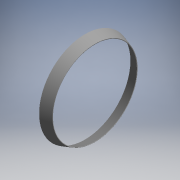
# Autodesk Inventor part: T4DB 170_cage
Saved by Autodesk Inventor 2017.3 (Build 213256000, 256)
## iProperties
Part Number: T4DB 170_cage
Material: Generic
Catalog Web Link: www.cadenas.de
Description: BT1_001_101_cage-Tapered roller bearings, single row
Vendor: SKF
Document SubType Name: Modeling
Designer: partserver
Manufacturer: SKF
Mass: 17.2348 g
Surface Area: 356.766 cm^2
Volume: 17.2348 cm^3
Density: 1 g/cm^3
Appearance: PSOLRGB-175-175-175
Category: PARTsolutions
Company: SKF
Title: T4DB 170_cage
Author: Cadenas PARTsolutions
Comments: Tapered roller bearings, single row
PSOL_IDENT_0: {$CADENAS_DATA\23d-libs\skf\bearings_units_and_housings\roller_bearings\tapered_roller_bearings\tape
PSOL_IDENT_1: red_roller_bearings_single_row\parts\bt1_001_101_cage.prj},178 {VTYP=3D},{NB=T4DB 170_cage},{LINA=T4
PSOL_IDENT_2: DB 170_cage},{NN=BT1_001_101_cage},{DATE=23.12.2020 07:01:43},{GEOMDATE=22.10.2020 06:54:36},{VERSIO
PSOL_IDENT_3: N=},{LINEID=4320},{WBVAR=},{WBNUMERIC=}  {NB=T4DB 170_cage},{LINA=T4DB 170_cage},{KT=DUMMY},{DESIGNA
PSOL_IDENT_4: TION=T4DB 170},{DD=170.000},{D=230.000},{T=32.000},{DD1=197.5000},{D1=MIN},{ALPHA=17.100},{RANGLE=2.
PSOL_IDENT_5: 500},{IRA=14.600},{B=30.000},{C=23.000},{C1=MIN},{R12=3.0},{R34=3.0},{AA=44.29541},{PITCH=200.033},{
PSOL_IDENT_6: DW=16.450},{LW=21.500},{DDAMAX=182},{DDAMIN=184.5},{DAMIN=215},{DAMAX=216.0},{DBMIN=223},{CA=6},{CB=
PSOL_IDENT_7: 9.0},{RA=3.0},{RB=3.0},{LOAD1=307.000},{LOAD2=440.000},{LOAD3=43.000},{SPEED1=2000},{SPEED2=2600},{E
PSOL_IDENT_8: E=0.46},{Y=1.30},{Y0=0.7},{Y1=0},{X1=1},{X2=0.4},{X0=0.5},{Z=37},{II=1},{R1=0.00000231},{R2=10.9},{S
PSOL_IDENT_9: 1=0.019},{S2=2},{KZ=6},{KL=0.7},{BF=2},{MASS=3.439},{DESIGN=trb1},{HELP=0.000},{PPATH=parts/bt1_001_
PSOL_IDENT_10: 101_asmtpl.prj},{SUPPRESS=N},{A4=200000},{A15=350000},{BEARING=T4DB 170},{A8=300000},{POPULAR=}
NB: T4DB 170_cage
NN: BT1_001_101_cage
NT: Tapered roller bearings, single row
NBSYN: $DESIGNATION._cage
LINA: T4DB 170_cage
CATALOG: SKF
DESIGNATION: T4DB 170
DD: 170
D: 230
T: 32
DD1: 197.5
D1: 0
ALPHA: 17.1
RANGLE: 2.5
IRA: 14.6
B: 30
C: 23
C1: 0
R12: 3
R34: 3
AA: 44.29541
PITCH: 200.033
DW: 16.45
LW: 21.5
DDAMAX: 182
DDAMIN: 184.5
DAMIN: 215
DAMAX: 216
DBMIN: 223
CA: 6
CB: 9
RA: 3
RB: 3
LOAD1: 307
LOAD2: 440
LOAD3: 43
SPEED1: 2000
SPEED2: 2600
EE: 0.46
Y: 1.3
Y0: 0.7
Y1: 0
X1: 1
X2: 0.4
X0: 0.5
Z: 37
II: 1
R1: 0.00000231
R2: 10.9
S1: 0.019
S2: 2
KZ: 6
KL: 0.7
BF: 2
MASS: 3.439
PPATH: parts/bt1_001_101_asmtpl.prj
SUPPRESS: N
A4: 200000
A15: 350000
BEARING: T4DB 170
A8: 300000
SUPPLIER: SKF
ARTICLENO: T4DB 170_cage
BOMINFO: T4DB 170_cage
CREATOR: CADENAS GmbH
Autodesk Inventor part; units mm, degrees
sketch "Sketch_1" plane through (0, 0, 0) normal (0, 0, 1) x (1, 0, 0)
  line L0 (50, 0) -> (-50, 0)
  arc A0 (-0.1653, 102.1585) -> (-0.3576, 101.7856) centre (-0.0709, 101.8738) ccw
  line L1 (-0.3576, 101.7856) -> (-0.0028, 100.6321)
  line L2 (-0.0028, 100.6321) -> (0.9466, 100.947)
  line L3 (0.9466, 100.947) -> (0.8571, 101.238)
  arc A1 (0.9853, 101.4866) -> (0.8571, 101.238) centre (1.0482, 101.2968) ccw
  line L4 (0.9853, 101.4866) -> (24.0593, 109.1399)
  line L5 (24.0593, 109.1399) -> (23.7652, 110.096)
  line L6 (23.7652, 110.096) -> (-0.1653, 102.1585)
  constraints: 14 end point, 4 point on circle, 2 centre point
revolve "Revolution1" add sketch "Sketch_1" angle 360 about axis through (50, 0, 0) along (1, 0, 0)
ref_plane "cage_XY" through (0, 0, 0) normal (0, 0, 1) x (1, 0, 0)
ref_plane "cage_YZ" through (0, 0, 0) normal (1, 0, 0) x (0, 1, 0)
ref_plane "cage_ZX" through (0, 0, 0) normal (0, 1, 0) x (0, 0, 1)
ref_plane "roller1_XY" through (0, 100.0165, 0) normal (1, 0, 0) x (0, 0, -1)
ref_plane "roller1_YZ" through (0, 100.0165, 0) normal (0, 0, -1) x (0, 1, 0)
ref_plane "roller1_ZX" through (0, 100.0165, 0) normal (0, 1, 0) x (1, 0, 0)
ref_plane "roller10_XY" through (0, 4.2448, 99.9264) normal (1, 0, 0) x (0, 0.9991, -0.0424)
ref_plane "roller10_YZ" through (0, 4.2448, 99.9264) normal (0, 0.9991, -0.0424) x (0, 0.0424, 0.9991)
ref_plane "roller10_ZX" through (0, 4.2448, 99.9264) normal (0, 0.0424, 0.9991) x (1, 0, 0)
ref_plane "roller11_XY" through (0, -12.7039, 99.2064) normal (1, 0, 0) x (0, 0.9919, 0.127)
ref_plane "roller11_YZ" through (0, -12.7039, 99.2064) normal (0, 0.9919, 0.127) x (0, -0.127, 0.9919)
ref_plane "roller11_ZX" through (0, -12.7039, 99.2064) normal (0, -0.127, 0.9919) x (1, 0, 0)
ref_plane "roller12_XY" through (0, -29.2871, 95.6325) normal (1, 0, 0) x (0, 0.9562, 0.2928)
ref_plane "roller12_YZ" through (0, -29.2871, 95.6325) normal (0, 0.9562, 0.2928) x (0, -0.2928, 0.9562)
ref_plane "roller12_ZX" through (0, -29.2871, 95.6325) normal (0, -0.2928, 0.9562) x (1, 0, 0)
ref_plane "roller13_XY" through (0, -45.0278, 89.3073) normal (1, 0, 0) x (0, 0.8929, 0.4502)
ref_plane "roller13_YZ" through (0, -45.0278, 89.3073) normal (0, 0.8929, 0.4502) x (0, -0.4502, 0.8929)
ref_plane "roller13_ZX" through (0, -45.0278, 89.3073) normal (0, -0.4502, 0.8929) x (1, 0, 0)
ref_plane "roller14_XY" through (0, -59.4731, 80.413) normal (1, 0, 0) x (0, 0.804, 0.5946)
ref_plane "roller14_YZ" through (0, -59.4731, 80.413) normal (0, 0.804, 0.5946) x (0, -0.5946, 0.804)
ref_plane "roller14_ZX" through (0, -59.4731, 80.413) normal (0, -0.5946, 0.804) x (1, 0, 0)
ref_plane "roller15_XY" through (0, -72.2075, 69.2053) normal (1, 0, 0) x (0, 0.6919, 0.722)
ref_plane "roller15_YZ" through (0, -72.2075, 69.2053) normal (0, 0.6919, 0.722) x (0, -0.722, 0.6919)
ref_plane "roller15_ZX" through (0, -72.2075, 69.2053) normal (0, -0.722, 0.6919) x (1, 0, 0)
ref_plane "roller16_XY" through (0, -82.8646, 56.0067) normal (1, 0, 0) x (0, 0.56, 0.8285)
ref_plane "roller16_YZ" through (0, -82.8646, 56.0067) normal (0, 0.56, 0.8285) x (0, -0.8285, 0.56)
ref_plane "roller16_ZX" through (0, -82.8646, 56.0067) normal (0, -0.8285, 0.56) x (1, 0, 0)
ref_plane "roller17_XY" through (0, -91.1379, 41.1969) normal (1, 0, 0) x (0, 0.4119, 0.9112)
ref_plane "roller17_YZ" through (0, -91.1379, 41.1969) normal (0, 0.4119, 0.9112) x (0, -0.9112, 0.4119)
ref_plane "roller17_ZX" through (0, -91.1379, 41.1969) normal (0, -0.9112, 0.4119) x (1, 0, 0)
ref_plane "roller18_XY" through (0, -96.7893, 25.202) normal (1, 0, 0) x (0, 0.252, 0.9677)
ref_plane "roller18_YZ" through (0, -96.7893, 25.202) normal (0, 0.252, 0.9677) x (0, -0.9677, 0.252)
ref_plane "roller18_ZX" through (0, -96.7893, 25.202) normal (0, -0.9677, 0.252) x (1, 0, 0)
ref_plane "roller19_XY" through (0, -99.6562, 8.482) normal (1, 0, 0) x (0, 0.0848, 0.9964)
ref_plane "roller19_YZ" through (0, -99.6562, 8.482) normal (0, 0.0848, 0.9964) x (0, -0.9964, 0.0848)
ref_plane "roller19_ZX" through (0, -99.6562, 8.482) normal (0, -0.9964, 0.0848) x (1, 0, 0)
ref_plane "roller2_XY" through (0, 98.5779, 16.9029) normal (1, 0, 0) x (0, 0.169, -0.9856)
ref_plane "roller2_YZ" through (0, 98.5779, 16.9029) normal (0, 0.169, -0.9856) x (0, 0.9856, 0.169)
ref_plane "roller2_ZX" through (0, 98.5779, 16.9029) normal (0, 0.9856, 0.169) x (1, 0, 0)
ref_plane "roller20_XY" through (0, -99.6562, -8.482) normal (1, 0, 0) x (0, -0.0848, 0.9964)
ref_plane "roller20_YZ" through (0, -99.6562, -8.482) normal (0, -0.0848, 0.9964) x (0, -0.9964, -0.0848)
ref_plane "roller20_ZX" through (0, -99.6562, -8.482) normal (0, -0.9964, -0.0848) x (1, 0, 0)
ref_plane "roller21_XY" through (0, -96.7893, -25.202) normal (1, 0, 0) x (0, -0.252, 0.9677)
ref_plane "roller21_YZ" through (0, -96.7893, -25.202) normal (0, -0.252, 0.9677) x (0, -0.9677, -0.252)
ref_plane "roller21_ZX" through (0, -96.7893, -25.202) normal (0, -0.9677, -0.252) x (1, 0, 0)
ref_plane "roller22_XY" through (0, -91.1379, -41.1969) normal (1, 0, 0) x (0, -0.4119, 0.9112)
ref_plane "roller22_YZ" through (0, -91.1379, -41.1969) normal (0, -0.4119, 0.9112) x (0, -0.9112, -0.4119)
ref_plane "roller22_ZX" through (0, -91.1379, -41.1969) normal (0, -0.9112, -0.4119) x (1, 0, 0)
ref_plane "roller23_XY" through (0, -82.8646, -56.0067) normal (1, 0, 0) x (0, -0.56, 0.8285)
ref_plane "roller23_YZ" through (0, -82.8646, -56.0067) normal (0, -0.56, 0.8285) x (0, -0.8285, -0.56)
ref_plane "roller23_ZX" through (0, -82.8646, -56.0067) normal (0, -0.8285, -0.56) x (1, 0, 0)
ref_plane "roller24_XY" through (0, -72.2075, -69.2053) normal (1, 0, 0) x (0, -0.6919, 0.722)
ref_plane "roller24_YZ" through (0, -72.2075, -69.2053) normal (0, -0.6919, 0.722) x (0, -0.722, -0.6919)
ref_plane "roller24_ZX" through (0, -72.2075, -69.2053) normal (0, -0.722, -0.6919) x (1, 0, 0)
ref_plane "roller25_XY" through (0, -59.4731, -80.413) normal (1, 0, 0) x (0, -0.804, 0.5946)
ref_plane "roller25_YZ" through (0, -59.4731, -80.413) normal (0, -0.804, 0.5946) x (0, -0.5946, -0.804)
ref_plane "roller25_ZX" through (0, -59.4731, -80.413) normal (0, -0.5946, -0.804) x (1, 0, 0)
ref_plane "roller26_XY" through (0, -45.0278, -89.3073) normal (1, 0, 0) x (0, -0.8929, 0.4502)
ref_plane "roller26_YZ" through (0, -45.0278, -89.3073) normal (0, -0.8929, 0.4502) x (0, -0.4502, -0.8929)
ref_plane "roller26_ZX" through (0, -45.0278, -89.3073) normal (0, -0.4502, -0.8929) x (1, 0, 0)
ref_plane "roller27_XY" through (0, -29.2871, -95.6325) normal (1, 0, 0) x (0, -0.9562, 0.2928)
ref_plane "roller27_YZ" through (0, -29.2871, -95.6325) normal (0, -0.9562, 0.2928) x (0, -0.2928, -0.9562)
ref_plane "roller27_ZX" through (0, -29.2871, -95.6325) normal (0, -0.2928, -0.9562) x (1, 0, 0)
ref_plane "roller28_XY" through (0, -12.7039, -99.2064) normal (1, 0, 0) x (0, -0.9919, 0.127)
ref_plane "roller28_YZ" through (0, -12.7039, -99.2064) normal (0, -0.9919, 0.127) x (0, -0.127, -0.9919)
ref_plane "roller28_ZX" through (0, -12.7039, -99.2064) normal (0, -0.127, -0.9919) x (1, 0, 0)
ref_plane "roller29_XY" through (0, 4.2448, -99.9264) normal (1, 0, 0) x (0, -0.9991, -0.0424)
ref_plane "roller29_YZ" through (0, 4.2448, -99.9264) normal (0, -0.9991, -0.0424) x (0, 0.0424, -0.9991)
ref_plane "roller29_ZX" through (0, 4.2448, -99.9264) normal (0, 0.0424, -0.9991) x (1, 0, 0)
ref_plane "roller3_XY" through (0, 94.3033, 33.3195) normal (1, 0, 0) x (0, 0.3331, -0.9429)
ref_plane "roller3_YZ" through (0, 94.3033, 33.3195) normal (0, 0.3331, -0.9429) x (0, 0.9429, 0.3331)
ref_plane "roller3_ZX" through (0, 94.3033, 33.3195) normal (0, 0.9429, 0.3331) x (1, 0, 0)
ref_plane "roller30_XY" through (0, 21.0714, -97.7717) normal (1, 0, 0) x (0, -0.9776, -0.2107)
ref_plane "roller30_YZ" through (0, 21.0714, -97.7717) normal (0, -0.9776, -0.2107) x (0, 0.2107, -0.9776)
ref_plane "roller30_ZX" through (0, 21.0714, -97.7717) normal (0, 0.2107, -0.9776) x (1, 0, 0)
ref_plane "roller31_XY" through (0, 37.2918, -92.8042) normal (1, 0, 0) x (0, -0.9279, -0.3729)
ref_plane "roller31_YZ" through (0, 37.2918, -92.8042) normal (0, -0.9279, -0.3729) x (0, 0.3729, -0.9279)
ref_plane "roller31_ZX" through (0, 37.2918, -92.8042) normal (0, 0.3729, -0.9279) x (1, 0, 0)
ref_plane "roller32_XY" through (0, 52.4394, -85.167) normal (1, 0, 0) x (0, -0.8515, -0.5243)
ref_plane "roller32_YZ" through (0, 52.4394, -85.167) normal (0, -0.8515, -0.5243) x (0, 0.5243, -0.8515)
ref_plane "roller32_ZX" through (0, 52.4394, -85.167) normal (0, 0.5243, -0.8515) x (1, 0, 0)
ref_plane "roller33_XY" through (0, 66.0784, -75.0796) normal (1, 0, 0) x (0, -0.7507, -0.6607)
ref_plane "roller33_YZ" through (0, 66.0784, -75.0796) normal (0, -0.7507, -0.6607) x (0, 0.6607, -0.7507)
ref_plane "roller33_ZX" through (0, 66.0784, -75.0796) normal (0, 0.6607, -0.7507) x (1, 0, 0)
ref_plane "roller34_XY" through (0, 77.8164, -62.8324) normal (1, 0, 0) x (0, -0.6282, -0.778)
ref_plane "roller34_YZ" through (0, 77.8164, -62.8324) normal (0, -0.6282, -0.778) x (0, 0.778, -0.6282)
ref_plane "roller34_ZX" through (0, 77.8164, -62.8324) normal (0, 0.778, -0.6282) x (1, 0, 0)
ref_plane "roller35_XY" through (0, 87.3158, -48.7775) normal (1, 0, 0) x (0, -0.4877, -0.873)
ref_plane "roller35_YZ" through (0, 87.3158, -48.7775) normal (0, -0.4877, -0.873) x (0, 0.873, -0.4877)
ref_plane "roller35_ZX" through (0, 87.3158, -48.7775) normal (0, 0.873, -0.4877) x (1, 0, 0)
ref_plane "roller36_XY" through (0, 94.3033, -33.3195) normal (1, 0, 0) x (0, -0.3331, -0.9429)
ref_plane "roller36_YZ" through (0, 94.3033, -33.3195) normal (0, -0.3331, -0.9429) x (0, 0.9429, -0.3331)
ref_plane "roller36_ZX" through (0, 94.3033, -33.3195) normal (0, 0.9429, -0.3331) x (1, 0, 0)
ref_plane "roller37_XY" through (0, 98.5779, -16.9029) normal (1, 0, 0) x (0, -0.169, -0.9856)
ref_plane "roller37_YZ" through (0, 98.5779, -16.9029) normal (0, -0.169, -0.9856) x (0, 0.9856, -0.169)
ref_plane "roller37_ZX" through (0, 98.5779, -16.9029) normal (0, 0.9856, -0.169) x (1, 0, 0)
ref_plane "roller4_XY" through (0, 87.3158, 48.7775) normal (1, 0, 0) x (0, 0.4877, -0.873)
ref_plane "roller4_YZ" through (0, 87.3158, 48.7775) normal (0, 0.4877, -0.873) x (0, 0.873, 0.4877)
ref_plane "roller4_ZX" through (0, 87.3158, 48.7775) normal (0, 0.873, 0.4877) x (1, 0, 0)
ref_plane "roller5_XY" through (0, 77.8164, 62.8324) normal (1, 0, 0) x (0, 0.6282, -0.778)
ref_plane "roller5_YZ" through (0, 77.8164, 62.8324) normal (0, 0.6282, -0.778) x (0, 0.778, 0.6282)
ref_plane "roller5_ZX" through (0, 77.8164, 62.8324) normal (0, 0.778, 0.6282) x (1, 0, 0)
ref_plane "roller6_XY" through (0, 66.0784, 75.0796) normal (1, 0, 0) x (0, 0.7507, -0.6607)
ref_plane "roller6_YZ" through (0, 66.0784, 75.0796) normal (0, 0.7507, -0.6607) x (0, 0.6607, 0.7507)
ref_plane "roller6_ZX" through (0, 66.0784, 75.0796) normal (0, 0.6607, 0.7507) x (1, 0, 0)
ref_plane "roller7_XY" through (0, 52.4394, 85.167) normal (1, 0, 0) x (0, 0.8515, -0.5243)
ref_plane "roller7_YZ" through (0, 52.4394, 85.167) normal (0, 0.8515, -0.5243) x (0, 0.5243, 0.8515)
ref_plane "roller7_ZX" through (0, 52.4394, 85.167) normal (0, 0.5243, 0.8515) x (1, 0, 0)
ref_plane "roller8_XY" through (0, 37.2918, 92.8042) normal (1, 0, 0) x (0, 0.9279, -0.3729)
ref_plane "roller8_YZ" through (0, 37.2918, 92.8042) normal (0, 0.9279, -0.3729) x (0, 0.3729, 0.9279)
ref_plane "roller8_ZX" through (0, 37.2918, 92.8042) normal (0, 0.3729, 0.9279) x (1, 0, 0)
ref_plane "roller9_XY" through (0, 21.0714, 97.7717) normal (1, 0, 0) x (0, 0.9776, -0.2107)
ref_plane "roller9_YZ" through (0, 21.0714, 97.7717) normal (0, 0.9776, -0.2107) x (0, 0.2107, 0.9776)
ref_plane "roller9_ZX" through (0, 21.0714, 97.7717) normal (0, 0.2107, 0.9776) x (1, 0, 0)
body "Solid1"
